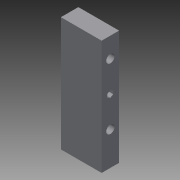
# Autodesk Inventor part: CNC-Y-axis- moving side to side plateform
Saved by Autodesk Inventor 2015 (Build 190159000, 159)
## iProperties
Created: 2015-03-24
Part Number: CNC-Y-axis- moving side to side plateform
Material: Generic
Document SubType Name: Modeling
Designer: Bangladesh
Density: 1 g/cm^3
Appearance: Default
Author: Bangladesh
Autodesk Inventor part; units mm, degrees
ref_plane "YZ Plane" through (0, 0, 0) normal (1, 0, 0) x (0, 1, 0)
ref_plane "XZ Plane" through (0, 0, 0) normal (0, 1, 0) x (-1, 0, 0)
ref_plane "XY Plane" through (0, 0, 0) normal (0, 0, 1) x (1, 0, 0)
sketch "Sketch4" plane through (0, 0, 0) normal (0, 1, 0) x (-1, 0, 0)
  line L0 (44.45, 19.05) -> (-44.45, 19.05)
  line L1 (-44.45, 19.05) -> (-44.45, -19.05)
  line L2 (-44.45, -19.05) -> (44.45, -19.05)
  line L3 (44.45, -19.05) -> (44.45, 19.05)
  line L4 (44.45, 19.05) -> (-44.45, -19.05) construction
  line L5 (-44.45, 19.05) -> (44.45, -19.05) construction
  point P0 (0, 0)
  dimension "d8" = 88.9
  dimension "d9" = 38.1
  constraints: 12 end point, 2 midpoint, 2 parallel, 1 horizontal, 1 perpendicular
  measures "d8" distance of L2.end L1.end
  measures "d9" distance of L0.end L1.end
extrude "Extrusion2" add sketch "Sketch4" along normal mid plane 250
sketch "Sketch5" plane through (44.45, -125, -19.05) normal (1, 0, 0) x (0, 0, -1)
  circle A0 centre (-19.05, 206.558) radius 9
  circle A1 centre (-19.05, 72.932) radius 9
  line L0 (-38.1, 250) -> (0, 250) projected
  circle A2 centre (-19.05, 139.745) radius 7.2555
  line L1 (-19.05, 132.4895) -> (-25.3334, 136.1172)
  line L2 (-25.3334, 136.1172) -> (-25.3334, 143.3727)
  line L3 (-25.3334, 143.3727) -> (-19.05, 147.0005)
  line L4 (-19.05, 147.0005) -> (-12.7666, 143.3727)
  line L5 (-12.7666, 143.3727) -> (-12.7666, 136.1173)
  line L6 (-12.7666, 136.1173) -> (-19.05, 132.4895)
  point P0 (-19.05, 125)
  dimension "d40" = 14.511
  dimension "d12" = 18
  dimension "d14" = 18
  dimension "d37" = 43.442
  dimension "d38" = 66.813
  dimension "d39" = 133.626
  dimension "d41" = 66.813
  constraints: 12 end point, 2 centre point, 1 coincident, 1 vertical alignment, 15 other
  measures "d12" diameter of A0
  measures "d14" diameter of A1
  measures "d37" distance from line of L0 A0.centre
  measures "d38" distance of point (-19.05, 139.745) A0.centre
  measures "d39" distance of A1.centre A0.centre
  measures "d41" distance of A1.centre point (-19.05, 139.745)
extrude "Extrusion4" cut sketch "Sketch5" against normal blind 103.1875 contours A0 | A1 | L5 L6 L1 L2 L3 L4
body "Solid2"
